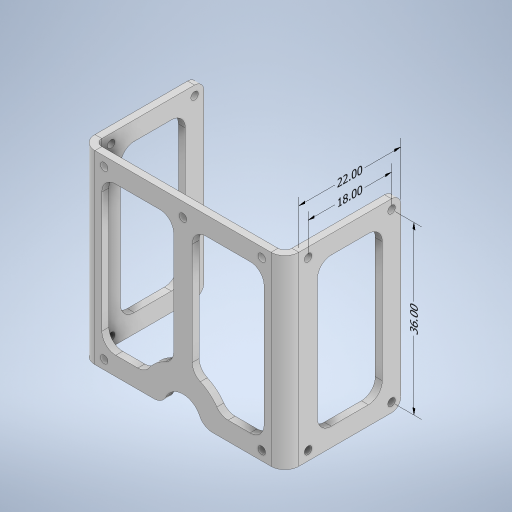
# Autodesk Inventor part: board_cover_top
Saved by Autodesk Inventor 2024.1 (Build 281209000, 209)
## iProperties
Created: 2024-02-15
Part Number: board_cover_top
Material: 一般
Document SubType Name: Sheet Metal
Designer: hibik
Density: 1 g/cm^3
Sheet Metal Rule: Default_mm
Appearance: 既定
Flat Pattern Width: 4 cm
Flat Pattern Length: 8.87858 cm
Flat Pattern Area: 35.5143 cm^2
Sheet Metal Width: 40.000 mm
Sheet Metal Length: 88.786 mm
Sheet Metal Area: 3551.434 mm^2
Author: hibik
Autodesk Inventor part; units mm, degrees
ref_plane "YZ Plane" through (0, 0, 0) normal (1, 0, 0) x (0, 1, 0)
ref_plane "XZ Plane" through (0, 0, 0) normal (0, 1, 0) x (-1, 0, 0)
ref_plane "XY Plane" through (0, 0, 0) normal (0, 0, 1) x (1, 0, 0)
sketch "スケッチ1" plane through (0, 0, 0) normal (0, 0, 1) x (1, 0, 0)
  line L0 (-22, 20) -> (22, 20)
  line L1 (22, 20) -> (22, -20)
  line L2 (22, -20) -> (-22, -20)
  line L3 (-22, -20) -> (-22, 20)
  line L4 (-22, 20) -> (22, -20) construction
  line L5 (22, 20) -> (-22, -20) construction
  point P0 (0, 0)
  dimension "d0" = 44
  dimension "d1" = 40
  measures "d0" distance of L1.end L2.end
  measures "d1" distance of L2.end L0.start
extrude "プレート1" add sketch "スケッチ1" along normal blind 1.5
sketch "スケッチ2" plane through (20.5, -20, 1.5) normal (1, 0, 0) x (0, 1, 0)
  line L0 (40, 0) -> (0, 0)
  line L1 (0, 0) -> (0, -25)
  line L2 (0, -25) -> (40, -25)
  line L3 (40, -25) -> (40, 0)
  constraints: 6 end point, 1 horizontal, 1 perpendicular, 1 vertical
edge flange "フランジ1" height 25 angle 90 thickness 1.5 bend radius 1.5 thickness toward (1, 0, 0) relief tear relief width 1.5 relief depth 0.75 corner gap 1.5 corner form 0 edges at (22, 0, 0) (-22, 0, 0) wall of the first edge with corners at (20.5, 20, 1.5) (20.5, -20, 1.5) (20.5, -20, -23.5) (20.5, 20, -23.5)
bend "曲げ1"
corner "コーナー1"
sketch "スケッチ3" plane through (22, -20, -23.5) normal (1, 0, 0) x (0, 0, -1)
  circle A0 centre (-2, 2) radius 2
  circle A1 centre (-2, 2) radius 0.8
  line L0 (0, 40) -> (0, 0) projected
  line L1 (0, 0) -> (-22, 0) projected
  arc A2 (-2, 0) -> (0, 2) centre (-2, 2) ccw
  line L2 (-2, 0) -> (0, 0)
  line L3 (-18, 36) -> (-4, 36)
  line L4 (-4, 36) -> (-4, 4)
  line L5 (-4, 4) -> (-18, 4)
  line L6 (-18, 4) -> (-18, 36)
  line L7 (-22, 40) -> (-22, 0) projected
  line L8 (-22, 40) -> (0, 40) projected
  line L9 (-22, 20) -> (0, 20) construction
  line L10 (-11, 40) -> (-11, 0) construction
  circle A3 centre (-20, 2) radius 0.8
  circle A4 centre (-2, 38) radius 0.8
  circle A5 centre (-20, 38) radius 0.8
  point P0 (-23.5, 20)
  dimension "d13" = 4
  dimension "d14" = 1.6
  dimension "d24" = 4
  dimension "d25" = 4
  dimension "d26" = 4
  dimension "d27" = 4
  constraints: 14 end point, 6 centre point, 4 midpoint, 4 point on circle, 3 symmetric about line, 2 horizontal, 2 parallel, 2 point on line, 2 tangent, 1 coincident, 1 concentric, 1 perpendicular, 3 other
  measures "d13" diameter of A0
  measures "d14" diameter of A1
  measures "d24" distance between parallel lines of L0 L4
  measures "d25" distance between parallel lines of L1 L5
  measures "d26" distance between parallel lines of L7 L6
  measures "d27" distance between parallel lines of L8 L3
extrude "切り取り1" cut sketch "スケッチ3" against normal blind 1.5 contours L0 L1 A0 | A1 | L3 L4 L5 L6 | A3 | A4 | A5
sketch "スケッチ4" plane through (0, 0, 1.5) normal (0, 0, 1) x (1, 0, 0)
  line L0 (-17.5, 16) -> (17.5, 16)
  line L1 (17.5, 16) -> (17.5, -16)
  line L2 (-17.5, -16) -> (-17.5, 16)
  line L3 (-17.5, 16) -> (17.5, -16) construction
  line L4 (17.5, 16) -> (-17.5, -16) construction
  line L5 (-19, -20) -> (19, -20) projected
  circle A0 centre (0, -20) radius 4
  circle A1 centre (0, -20) radius 9
  line L6 (17.5, -16) -> (8.0623, -16)
  line L7 (-8.0623, -16) -> (-17.5, -16)
  line L8 (-2, 16) -> (2, 16)
  line L9 (2, 16) -> (2, -11.225)
  line L10 (2, -11.225) -> (-2, -11.225)
  line L11 (-2, -11.225) -> (-2, 16)
  point P0 (0, 0)
  dimension "d17" = 35
  dimension "d18" = 32
  dimension "d19" = 5
  dimension "d22" = 4
  constraints: 22 end point, 5 parallel, 4 point on circle, 3 midpoint, 2 centre point, 2 horizontal, 2 perpendicular, 2 tangent, 1 coincident, 1 point on line
  measures "d17" distance of L0.start L0.end
  measures "d18" distance of L2.start L0.start
  measures "d19" radial gap between concentric circles of A1 A0
  measures "d22" distance of L9.end L10.end
extrude "切り取り2" cut sketch "スケッチ4" against normal blind 1.5 contours L0 L11 A1 L7 L2 | L0 L1 L6 A1 L9 | A0 L5 | L5 A0
fillet "フィレット1" radius 3 16 edges at (2, 16, 0.75) (17.5, 16, 0.75) (17.5, -16, 0.75) (8.0623, -16, 0.75) (2, -11.225, 0.75) (-2, -11.225, 0.75) (-8.0623, -16, 0.75) (-2, 16, 0.75) (-17.5, 16, 0.75) (-17.5, -16, 0.75) (4, -20, 0.75) (-4, -20, 0.75) (21.25, 16, -19.5) (21.25, 16, -5.5) (21.25, -16, -5.5) (21.25, -16, -19.5)
sketch "スケッチ6" plane through (0, 0, 1.5) normal (0, 0, 1) x (1, 0, 0)
  circle A0 centre (0, 17) radius 0.8
  circle A1 centre (0, -13) radius 0.8
  line L0 (-19, 20) -> (19, 20) projected
  arc A2 (3.614, -18.2857) -> (-3.614, -18.2857) centre (0, -20) ccw projected
  circle A3 centre (-17, 18) radius 0.8
  circle A4 centre (17, 18) radius 0.8
  line L1 (-10.0831, 0) -> (9.9169, 0)
  circle A5 centre (-17, -18) radius 0.8
  circle A6 centre (17, -18) radius 0.8
  point P0 (0, 0)
  dimension "d28" = 1.6
  dimension "d29" = 1.6
  dimension "d30" = 3
  dimension "d31" = 7
  dimension "d32" = 1.6
  dimension "d33" = 1.6
  dimension "d34" = 2
  dimension "d35" = 17
  dimension "d36" = 17
  constraints: 6 centre point, 2 end point, 2 symmetric about line, 2 vertical alignment, 1 horizontal, 1 horizontal alignment, 1 point on line, 2 other
  measures "d28" diameter of A0
  measures "d29" diameter of A1
  measures "d30" distance from line of L0 A0.centre
  measures "d31" distance of A2.centre A1.centre
  measures "d32" diameter of A3
  measures "d33" diameter of A4
  measures "d34" distance from line of L0 A4.centre
  measures "d35" horizontal distance of A0.centre A3.centre
  measures "d36" horizontal distance of A4.centre A0.centre
extrude "切り取り3" cut sketch "スケッチ6" against normal blind 1.5 contours A0 | A3 | A4 | A5 | A6
sketch "スケッチ7" plane through (-22, -20, -23.5) normal (-1, 0, 0) x (0, 0, 1)
  arc A0 (0, 2) -> (2, 0) centre (2, 2) ccw projected
  line L0 (0, 40) -> (0, 2) projected
  line L1 (22, 40) -> (0, 40) projected
  line L2 (22, 40) -> (22, 0) projected
  line L3 (2, 0) -> (22, 0) projected
  circle A1 centre (2, 38) radius 0.8 projected
  circle A2 centre (20, 2) radius 0.8 projected
  circle A3 centre (2, 2) radius 0.8 projected
  circle A4 centre (20, 38) radius 0.8 projected
  line L4 (18, 7) -> (18, 33) projected
  arc A5 (18, 33) -> (15, 36) centre (15, 33) ccw projected
  line L5 (15, 36) -> (7, 36) projected
  arc A6 (7, 36) -> (4, 33) centre (7, 33) ccw projected
  line L6 (4, 33) -> (4, 7) projected
  arc A7 (4, 7) -> (7, 4) centre (7, 7) ccw projected
  line L7 (7, 4) -> (15, 4) projected
  arc A8 (15, 4) -> (18, 7) centre (15, 7) ccw projected
  line L8 (22, 0) -> (22, 40) projected
  line L9 (0, 40) -> (22, 40) projected
  line L10 (0, 0) -> (0, 40) projected
  line L11 (22, 0) -> (0, 0) projected
  point P0 (23.5, 20)
extrude "切り取り4" cut sketch "スケッチ7" against normal blind 1.5 contours A0 L11 L10 | A1 | A2 | A3 | A4 | A8 L7 A7 L6 A6 L5 A5 L4
fillet "フィレット2" radius 2 2 edges at (-21.25, 20, -23.5) (21.25, 20, -23.5)
equation "\"d15\" = Thickness"
equation "\"d20\" = Thickness"
equation "\"d37\" = Thickness"
equation "\"d39\" = Thickness"
equation "\"d2\" = Thickness"
equation "\"d3\" = BendReliefWidth"
equation "\"d4\" = BendReliefDepth"
equation "\"d5\" = MinimumRemnant"
equation "\"d6\" = TransitionRadius"
equation "\"d9\" = BendRadius"
equation "\"d10\" = CornerReliefSize"
equation "\"d11\" = GapSize"
equation "\"d12\" = JacobiRadiusSize"
equation "\"BendRadius\" = Thickness"
equation "\"BendReliefWidth\" = Thickness"
equation "\"BendReliefDepth\" = 0.5 * Thickness"
equation "\"CornerReliefSize\" = 4 * Thickness"
equation "\"MinimumRemnant\" = 2 * Thickness"
equation "\"TransitionRadius\" = BendRadius"
equation "\"JacobiRadiusSize\" = BendRadius"
equation "\"GapSize\" = Thickness"
equation "\"Thickness\" = 1.5"
